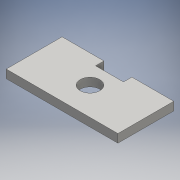
# Autodesk Inventor part: acople 2
Saved by Autodesk Inventor 2016 (Build 200138000, 138)
## iProperties
Created: 2016-08-02
Part Number: acople 2
Material: Genérico
Document SubType Name: Modeling
Designer: DanielFelipe
Density: 1 g/cm^3
Appearance: Valor por defecto
Author: DanielFelipe
Autodesk Inventor part; units mm, degrees
ref_plane "YZ Plane" through (0, 0, 0) normal (1, 0, 0) x (0, 1, 0)
ref_plane "XZ Plane" through (0, 0, 0) normal (0, 1, 0) x (-1, 0, 0)
ref_plane "XY Plane" through (0, 0, 0) normal (0, 0, 1) x (1, 0, 0)
sketch "Boceto1" plane through (0, 0, 0) normal (0, 0, 1) x (1, 0, 0)
  line L0 (-20, -10) -> (20, -10)
  line L1 (20, -10) -> (20, 10)
  line L2 (20, 10) -> (-20, 10)
  line L3 (-20, 10) -> (-20, -10)
  arc A0 (14, -2) -> (14, 2) centre (14, 0) ccw
  arc A1 (-2.4791, -2.4706) -> (2.4791, -2.4706) centre (0, 0) ccw
  arc A2 (-14, 2) -> (-14, -2) centre (-14, 0) ccw
  arc A3 (2.4791, 2.4706) -> (-2.4791, 2.4706) centre (0, 0) ccw
  circle A4 centre (0, 0) radius 3.5
  constraints: 8 end point, 8 point on circle, 5 centre point, 1 coincident, 1 concentric
extrude "Extrusión1" add sketch "Boceto1" along normal blind 3
sketch "Boceto2" plane through (0, 0, 3) normal (0, 0, 1) x (1, 0, 0)
  circle A0 centre (0, 0) radius 3.5 projected
  line L0 (-20, -10) -> (20, -10) projected
  line L1 (20, -10) -> (20, 10) projected
  line L2 (-20, 10) -> (-20, -10) projected
  line L3 (0, 7) -> (5, 7)
  line L4 (5, 7) -> (5, 10)
  line L5 (0, 7) -> (-5, 7)
  line L6 (-5, 7) -> (-5, 10)
  line L7 (-5, 7) -> (5, 7)
  line L8 (5, 7) -> (5, 10)
  line L9 (5, 10) -> (-5, 10)
  line L10 (-5, 10) -> (-5, 7)
  line L11 (-5, 7) -> (5, 7)
  line L12 (5, 7) -> (5, 17.8116)
  line L13 (5, 17.8116) -> (-5, 17.8116)
  line L14 (-5, 17.8116) -> (-5, 7)
  dimension "d3" = 5
  dimension "d4" = 5
  constraints: 24 end point, 4 parallel, 3 perpendicular, 2 horizontal, 1 centre point, 1 point on line
  measures "d3" distance of L3.start L3.end
  measures "d4" distance of L3.start L5.end
extrude "Extrusión2" cut sketch "Boceto2" against normal blind 3 contours L5 L6 L9 L4 L3
